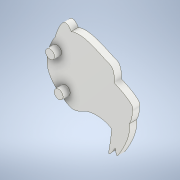
# Autodesk Inventor part: Component18
Saved by Autodesk Inventor 2022 (Build 260153000, 153)
## iProperties
Created: 2022-01-29
Part Number: Component18
Material: Generic
Document SubType Name: Modeling
Designer: Administrator
Density: 1 g/cm^3
Appearance: Default
Title: Component18
Author: Administrator
Autodesk Inventor part; units mm, degrees
ref_plane "YZ Plane" through (0, 0, 0) normal (1, 0, 0) x (0, 1, 0)
ref_plane "XZ Plane" through (0, 0, 0) normal (0, 1, 0) x (-1, 0, 0)
ref_plane "XY Plane" through (0, 0, 0) normal (0, 0, 1) x (1, 0, 0)
sketch "Sketch2" plane through (0, 0, 0) normal (0, 0, 1) x (1, 0, 0)
  circle A0 centre (-28.9423, -25.0501) radius 3.175
  circle A1 centre (-35.0338, -3.4521) radius 3.175
  spline S0 degree 5 poles (-36.4631, 3.8342) (-37.0372, 2.99) (-38.3286, 0.9192) (-40.0796, -2.5457) (-41.7868, -7.4597) (-42.601, -13.4201) (-41.8077, -18.9083) (-39.1083, -23.7876) (-34.9506, -28.0634) (-30.265, -31.4842) (-26.9371, -33.2868) (-25.0772, -33.9828) (-24.1731, -34.1374) (-23.8049, -34.1374) knots 0 0 0 0 0 0 0.083204 0.197804 0.312403 0.427003 0.541602 0.656202 0.770801 0.885401 1 1 1 1 1 1 weights 1 1 1 1 1 1 1 1 1 1 1 1 1 1
  spline S1 degree 5 poles (-23.8049, -34.1374) (-23.1085, -34.1374) (-21.8007, -34.0417) (-20.094, -33.6107) (-18.1733, -32.5618) (-15.5862, -30.9902) (-12.1545, -29.7446) (-7.5717, -29.2998) (-2.7747, -29.7298) (0.1536, -30.5342) (1.7933, -31.3237) (2.7949, -31.9218) (3.3555, -32.274) (3.4971, -32.3637) knots 0 0 0 0 0 0 0.1 0.2 0.3 0.4 0.5 0.6 0.7 0.8 0.833862 0.833862 0.833862 0.833862 0.833862 0.833862 weights 1 1 1 1 1 1 1 1 1 1 1 1 1 1
  spline S2 degree 5 poles (3.4971, -32.3637) (3.5002, -33.0044) (3.4749, -34.3218) (3.3423, -36.4061) (2.9963, -39.3438) (2.4108, -42.9443) (1.8492, -46.0444) (1.5232, -48.2112) (1.6279, -49.1191) (2.3783, -48.6103) (3.851, -46.8752) (5.3188, -44.712) (6.1479, -43.0801) (6.1178, -42.8451) (6.434, -44.4674) (7.0222, -46.6225) (7.4149, -47.5662) (7.9804, -46.9195) (9.1686, -45.0294) (10.8799, -42.0339) (12.8702, -38.2285) (14.7426, -33.9155) (16.0318, -29.6888) (16.4901, -26.5609) (16.4862, -24.5415) (16.3714, -23.4207) (16.3036, -22.9743) knots 0 0 0 0 0 0 0.04 0.08 0.12 0.16 0.2 0.24 0.28 0.32 0.36 0.4 0.44 0.48 0.52 0.56 0.6 0.64 0.68 0.72 0.76 0.8 0.84 0.869987 0.869987 0.869987 0.869987 0.869987 0.869987 weights 1 1 1 1 1 1 1 1 1 1 1 1 1 1 1 1 1 1 1 1 1 1 1 1 1 1 1
  spline S3 degree 5 poles (16.3036, -22.9743) (16.7327, -22.1548) (17.615, -20.2387) (18.2797, -17.8156) (18.1655, -15.7115) (17.9193, -14.375) (18.8461, -13.3689) (19.2135, -11.4597) (14.9343, -7.9469) (9.1312, -4.7607) (5.2538, -3.3102) (5.765, -3.6714) (5.9665, -0.5173) (4.9391, 4.2112) (3.4741, 6.2623) (1.2952, 6.8525) (-2.2375, 8.3862) (-7.0032, 10.6465) (-12.7354, 13.0275) (-17.7001, 14.0796) (-21.4041, 13.9585) (-23.8063, 13.4368) (-24.9847, 13.0661) (-24.9865, 13.0655) knots -0.954926 -0.954926 -0.954926 -0.954926 -0.954926 -0.954926 -0.933333 -0.9 -0.866667 -0.833333 -0.8 -0.766667 -0.733333 -0.7 -0.666667 -0.633333 -0.6 -0.566667 -0.533333 -0.5 -0.466667 -0.433333 -0.4 -0.366667 -0.366616 -0.366616 -0.366616 -0.366616 -0.366616 -0.366616 weights 1 1 1 1 1 1 1 1 1 1 1 1 1 1 1 1 1 1 1 1 1 1 1 1
  spline S4 degree 5 poles (-24.9865, 13.0655) (-25.1058, 13.2533) (-25.4838, 13.8289) (-26.1176, 14.6902) (-27.0018, 15.6406) (-28.1279, 16.3695) (-29.3715, 16.5019) (-30.5955, 15.9227) (-31.8007, 14.6591) (-32.9888, 12.7711) (-34.1615, 10.3234) (-35.0886, 7.9615) (-35.7781, 5.9787) (-36.2352, 4.5644) (-36.4631, 3.8342) knots 0.053969 0.053969 0.053969 0.053969 0.053969 0.053969 0.1 0.2 0.3 0.4 0.5 0.6 0.7 0.8 0.9 1 1 1 1 1 1 weights 1 1 1 1 1 1 1 1 1 1 1 1 1 1 1
  point P0 (0, 0)
  point P1 (29.9895, -33.8036)
  constraints: 2 centre point, 10 other
extrude "Extrusion1" add sketch "Sketch2" against normal blind 5 contours A0 | A1 | S4 S3 S2 S1 S0
extrude "Extrusion2" add sketch "Sketch2" along normal blind 5 contours A0 | A1
body "Solid1"
